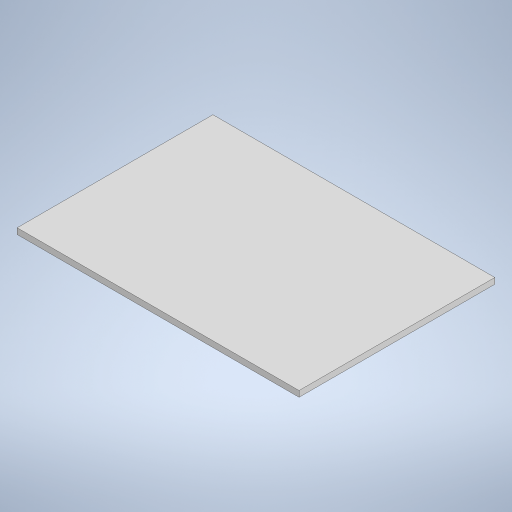
# Autodesk Inventor part: Tapa
Saved by Autodesk Inventor 2024 (Build 280153000, 153)
## iProperties
Created: 2023-07-29
Part Number: Tapa
Material: Genérico
Document SubType Name: Modeling
Designer: Det-Pc
Density: 1 g/cm^3
Appearance: Valor por defecto
Author: Det-Pc
Autodesk Inventor part; units mm, degrees
ref_plane "YZ Plane" through (0, 0, 0) normal (1, 0, 0) x (0, 1, 0)
ref_plane "XZ Plane" through (0, 0, 0) normal (0, 1, 0) x (-1, 0, 0)
ref_plane "XY Plane" through (0, 0, 0) normal (0, 0, 1) x (1, 0, 0)
sketch "Boceto1" plane through (0, 0, 0) normal (0, 1, 0) x (-1, 0, 0)
  line L0 (36, 25) -> (-36, 25)
  line L1 (-36, 25) -> (-36, -25)
  line L2 (-36, -25) -> (36, -25)
  line L3 (36, -25) -> (36, 25)
  point P0 (0, 0)
  point P1 (36, 0)
  point P2 (0, -25)
  dimension "d0" = 72
  dimension "d1" = 50
  constraints: 8 end point, 2 midpoint, 2 parallel, 1 horizontal, 1 horizontal alignment, 1 perpendicular, 1 vertical alignment
  measures "d0" distance of L0.start L0.end
  measures "d1" distance of L0.end L1.end
extrude "Extrusión1" add sketch "Boceto1" along normal blind 1.5
